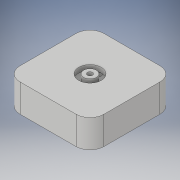
# Autodesk Inventor part: Unit_v3
Saved by Autodesk Inventor 2019 (Build 230136000, 136)
## iProperties
Created: 2018-11-21
Part Number: Unit_v3
Material: Generic
Document SubType Name: Modeling
Designer: Jeffrey Tan
Density: 1 g/cm^3
Appearance: Default
Author: Jeffrey Tan
Autodesk Inventor part; units mm, degrees
ref_plane "YZ Plane" through (0, 0, 0) normal (1, 0, 0) x (0, 1, 0)
ref_plane "XZ Plane" through (0, 0, 0) normal (0, 1, 0) x (-1, 0, 0)
ref_plane "XY Plane" through (0, 0, 0) normal (0, 0, 1) x (1, 0, 0)
sketch "Sketch1" plane through (0, 0, 0) normal (0, 1, 0) x (-1, 0, 0)
  line L0 (9.525, 9.525) -> (-9.525, 9.525)
  line L1 (-9.525, 9.525) -> (-9.525, -9.525)
  line L2 (-9.525, -9.525) -> (9.525, -9.525)
  line L3 (9.525, -9.525) -> (9.525, 9.525)
  point P0 (0, 0)
  dimension "d0" = 19.05
  dimension "d1" = 19.05
  dimension "d2" = 9.525
  dimension "d3" = 9.525
  constraints: 8 end point, 2 parallel, 1 horizontal, 1 perpendicular
  measures "d0" distance of L0.start L0.end
  measures "d1" distance of L0.end L1.end
  measures "d2" distance from line of point (0, 0) L1
  measures "d3" distance from line of L0 point (0, 0)
extrude "Extrusion1" add sketch "Sketch1" along normal blind 6.35
sketch "Sketch2" plane through (0, 6.35, 0) normal (0, 1, 0) x (1, 0, 0)
  circle A0 centre (0, 0) radius 1.4288
  circle A1 centre (0, 0) radius 2.5717
  circle A2 centre (0, 0) radius 0.5715
  dimension "d6" = 2.8575
  dimension "d7" = 5.1435
  dimension "d8" = 1.143
  constraints: 3 centre point, 3 coincident
  measures "d6" diameter of A0
  measures "d7" diameter of A1
  measures "d8" diameter of A2
extrude "Extrusion2" cut sketch "Sketch2" against normal blind 1.143 contours A1
extrude "Extrusion3" cut sketch "Sketch2" against normal through all contours A2
sketch "Sketch3" plane through (0, 5.207, 0) normal (0, 1, 0) x (1, 0, 0)
  circle A0 centre (0, 2.0003) radius 0.5715
  line L0 (0, 2.0003) -> (0, 0)
  dimension "d13" = 1.143
  dimension "d14" = 2.0002
  constraints: 2 end point, 1 centre point, 1 vertical
  measures "d13" diameter of A0
  measures "d14" distance of L0.end L0.start
extrude "Extrusion4" cut sketch "Sketch3" against normal through all
fillet "Fillet1" radius 3.175 4 edges at (-9.525, 3.175, 9.525) (9.525, 3.175, 9.525) (9.525, 3.175, -9.525) (-9.525, 3.175, -9.525)
body "Solid1"
